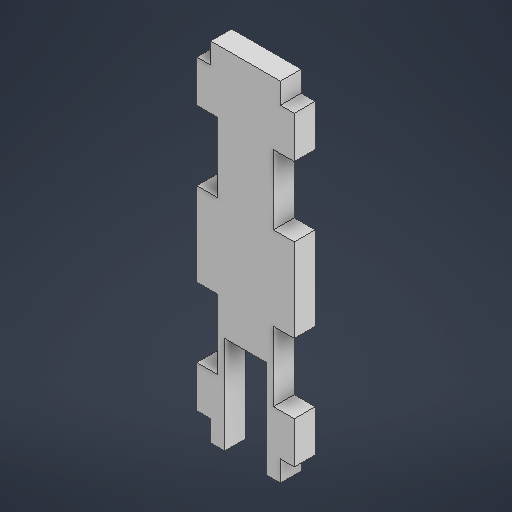
# Autodesk Inventor part: columna_techoV2
Saved by Autodesk Inventor 2026 (Build 300175000, 175)
## iProperties
Created: 2026-05-15
Part Number: columna_techoV2
Material: Generic
Document SubType Name: Modeling
Designer: juana
Density: 1 g/cm^3
Appearance: Default
Author: juana
Autodesk Inventor part; units mm, degrees
ref_plane "YZ Plane" through (0, 0, 0) normal (1, 0, 0) x (0, 1, 0)
ref_plane "XZ Plane" through (0, 0, 0) normal (0, 1, 0) x (-1, 0, 0)
ref_plane "XY Plane" through (0, 0, 0) normal (0, 0, 1) x (1, 0, 0)
sketch "Sketch1" plane through (0, 0, 0) normal (0, 0, 1) x (1, 0, 0)
  line L0 (0, 50) -> (14, 50)
  line L1 (14, 50) -> (14, 0)
  line L2 (14, 0) -> (0, 0)
  line L3 (0, 0) -> (0, 50)
  line L4 (2, 0) -> (12, 0)
  line L5 (12, 0) -> (12, 3)
  line L6 (2, 3) -> (2, 0)
  line L7 (0, 25) -> (14, 25) construction
  line L8 (12, 50) -> (12, 47)
  line L9 (2, 47) -> (2, 50)
  line L10 (2, 3) -> (0, 3)
  line L11 (12, 3) -> (14, 3)
  line L12 (2, 47) -> (0, 47)
  line L13 (12, 47) -> (14, 47)
  line L14 (14, 9) -> (11, 9)
  line L15 (11, 9) -> (11, 19)
  line L16 (11, 19) -> (14, 19)
  line L17 (14, 19) -> (14, 9)
  line L18 (0, 25) -> (14, 25) construction
  line L19 (14, 25) -> (14, 3) construction
  line L20 (14, 3) -> (0, 3) construction
  line L21 (0, 3) -> (0, 25) construction
  line L22 (7, 25) -> (7, 3) construction
  line L23 (0, 9) -> (3, 9)
  line L24 (3, 9) -> (3, 19)
  line L25 (3, 19) -> (0, 19)
  line L26 (14, 41) -> (11, 41)
  line L27 (11, 41) -> (11, 31)
  line L28 (11, 31) -> (14, 31)
  line L29 (0, 41) -> (3, 41)
  line L30 (3, 41) -> (3, 31)
  line L31 (3, 31) -> (0, 31)
  point P0 (7, 0)
  point P1 (14, 14)
  point P2 (11, 14)
  dimension "d0" = 14
  dimension "d1" = 10
  dimension "d3" = 3
  dimension "d4" = 50
  dimension "d5" = 5
  dimension "d6" = 10
  dimension "d7" = 3
  constraints: 64 end point, 16 symmetric about line, 8 point on line, 7 parallel, 7 perpendicular, 6 midpoint, 4 horizontal, 4 horizontal alignment, 1 coincident, 1 vertical alignment
  measures "d0" distance of L1.end L2.end
  measures "d1" distance of L5.end L6.start
  measures "d3" distance of L6.start L4.start
  measures "d4" distance of L2.end L0.start
  measures "d5" distance from line of L6 L22.end
  measures "d6" distance of L14.end L15.end
  measures "d7" distance of L15.end L16.end
extrude "Extrusion1" add sketch "Sketch1" along normal blind 3 contours L0 L8 L13 L1 L26 L27 L28 L16 L15 L14 L11 L5 L2 L6 L10 L3 L23 L24 L25 L31 L30 L29 L12 L9
sketch "Sketch2" plane through (0, 0, 3) normal (0, 0, 1) x (1, 0, 0)
  line L0 (4, 14) -> (10, 14)
  line L1 (10, 14) -> (10, 0)
  line L2 (10, 0) -> (4, 0)
  line L3 (4, 0) -> (4, 14)
  line L4 (2, 0) -> (12, 0) construction
  line L5 (3, 19) -> (3, 9) construction
  point P0 (0, 0)
  point P1 (7, 0)
  point P2 (7, 0)
  point P3 (3, 14)
  dimension "d10" = 6
  constraints: 8 end point, 3 midpoint, 2 horizontal alignment, 2 parallel, 1 coincident, 1 horizontal, 1 perpendicular
  measures "d10" distance of L0.start L0.end
extrude "Extrusion2" cut sketch "Sketch2" against normal blind 10
body "Solid1"
